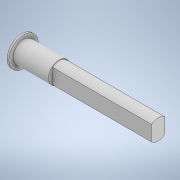
# Autodesk Inventor part: wielas
Saved by Autodesk Inventor 2022 (Build 260153000, 153)
## iProperties
Created: 2021-12-21
Part Number: wielas
Material: Generic
Document SubType Name: Modeling
Designer: keemi
Density: 1 g/cm^3
Appearance: Default
Author: keemi
Autodesk Inventor part; units mm, degrees
ref_plane "YZ Plane" through (0, 0, 0) normal (1, 0, 0) x (0, 1, 0)
ref_plane "XZ Plane" through (0, 0, 0) normal (0, 1, 0) x (-1, 0, 0)
ref_plane "XY Plane" through (0, 0, 0) normal (0, 0, 1) x (1, 0, 0)
sketch "Sketch1" plane through (0, 0, 0) normal (1, 0, 0) x (0, 1, 0)
  circle A0 centre (0, 0) radius 4
  dimension "d0" = 8
  constraints: 1 centre point, 1 coincident
  measures "d0" diameter of A0
extrude "Extrusion1" add sketch "Sketch1" along normal blind 0.5
sketch "Sketch2" plane through (0.5, 0, 0) normal (1, 0, 0) x (0, 0, -1)
  circle A0 centre (0, 0) radius 2.9
  circle A1 centre (0, 0) radius 2.75
  line L0 (0, 0) -> (-1.8, 0)
  line L1 (-1.8, 0) -> (-1.8, 3.3564)
  line L2 (-1.8, 3.3564) -> (0, 3.3564)
  line L3 (0, 3.3564) -> (0, 0)
  line L4 (-1.8, 3.3564) -> (1.8, 3.3564)
  line L5 (1.8, 3.3564) -> (1.8, -4.1498)
  line L6 (1.8, -4.1498) -> (-1.8, -4.1498)
  line L7 (-1.8, -4.1498) -> (-1.8, 3.3564)
  dimension "d3" = 5.8
  dimension "d6" = 5.5
  dimension "d7" = 1.8
  dimension "d8" = 3.6
  constraints: 16 end point, 4 parallel, 2 centre point, 2 coincident, 2 horizontal, 2 perpendicular
  measures "d3" diameter of A0
  measures "d6" diameter of A1
  measures "d7" distance of L1.end L2.end
  measures "d8" distance of L5.end L6.end
extrude "Extrusion2" add sketch "Sketch2" along normal blind 9.7 contours A0 L5 A1 | L5 A1 L3 A0 | A0 L7 A1 L5 | L3 A1 L1 A0 | L5 A1 L7 L0 L3 | A1 L5 | A0 L1 A1 L7 | L3 L0 L1 A1 | A1 L1 L7
sketch "Sketch3" plane through (10.2, 0, 0) normal (1, 0, 0) x (0, 0, -1)
  circle A0 centre (0, 0) radius 2.75
  line L0 (0, 0) -> (-1.8, 0)
  line L1 (-1.8, 0) -> (-1.8, 4.5353)
  line L2 (-1.8, 4.5353) -> (1.8, 4.5353)
  line L3 (1.8, 4.5353) -> (1.8, -4.8197)
  line L4 (1.8, -4.8197) -> (-1.8, -4.8197)
  line L5 (-1.8, -4.8197) -> (-1.8, 4.5353)
  point P0 (-1.8, -2.0791)
  point P1 (1.8, -2.0791)
  point P2 (1.8, 2.0791)
  point P3 (-1.8, 2.0791)
  dimension "d9" = 5.5
  dimension "d10" = 1.8
  dimension "d11" = 3.6
  constraints: 12 end point, 2 horizontal, 2 parallel, 1 centre point, 1 coincident, 1 perpendicular, 1 vertical
  measures "d9" diameter of A0
  measures "d10" distance of L0.start L0.end
  measures "d11" distance of L3.end L4.end
extrude "Extrusion3" add sketch "Sketch3" along normal blind 27 contours L3 A0 L5 L1
body "Solid1"
